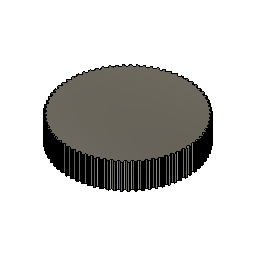
gear_75z (Autodesk Fusion 360 design; units mm, degrees)
Autodesk Fusion 360 part; units mm, degrees
sketch "Sketch1" plane through (0, 0, 0) normal (0, 0, 1) x (1, 0, 0) in component "gt2 pulley"
  circle A0 centre (0, 0) radius 23.8732 construction
  circle A1 centre (0, 0) radius 22.8692 construction
  line L0 (0, 0) -> (0, 23.8732) construction
  line L1 (0, 0) -> (0.9997, 23.8523) construction
  line L2 (0, 0) -> (1.4052, 23.8319) construction
  circle A2 centre (0, 0) radius 23.6192 construction
  arc A3 (0.3948, 23.4823) -> (0.4704, 23.1859) centre (1.3902, 23.5783) ccw
  circle A4 centre (0, 0) radius 23.4692 construction
  arc A5 (0.247, 23.6179) -> (0, 23.6192) centre (0, 0) ccw
  arc A6 (0.3948, 23.4823) -> (0.247, 23.6179) centre (0.2455, 23.468) ccw
  arc A7 (0.4704, 23.1859) -> (0.9577, 22.8492) centre (0.9809, 23.4037) ccw
  arc A8 (0, 23.6192) -> (-0.247, 23.6179) centre (0, 0) ccw
  arc A9 (-0.247, 23.6179) -> (-0.3948, 23.4823) centre (-0.2455, 23.468) ccw
  arc A10 (-0.4704, 23.1859) -> (-0.3948, 23.4823) centre (-1.3902, 23.5783) ccw
  arc A11 (-0.9577, 22.8492) -> (-0.4704, 23.1859) centre (-0.9809, 23.4037) ccw
  arc A12 (0.9577, 22.8492) -> (-0.9577, 22.8492) centre (0, 0) ccw
  point P0 (1.3902, 23.5783)
  point P1 (0, 23.6192)
  dimension "d18" = 47.7465
  dimension "d19" = 2.4
  dimension "d22" = 1.004
  dimension "d24" = 0.75
  dimension "d26" = 1
  dimension "d27" = 0.15
  dimension "d28" = 0.15
  dimension "d47" = 0.555
  dimension "d52" = 3.812
  constraint coincident A0.centre A1.centre
  constraint coincident A0 L0.end
  constraint vertical L0
  constraint coincident A0 L1.end
  constraint coincident A0 L2.end
  constraint concentric A1 A2
  constraint coincident A1 A7.end
  constraint coincident L1 A7.end
  constraint coincident A2 P0
  constraint coincident L2 P0
  constraint coincident P0 A3.centre
  constraint coincident A2 P1
  constraint coincident L0 P1
  constraint concentric A2 A4
  constraint coincident P1 A5.end
  constraint coincident A4 A6.centre
  constraint coincident A3.start A6.start
  constraint tangent A3 A6
  constraint tangent A3 A7
  constraint symmetric L0 A7.end A11.start
  constraint symmetric L0 A3.start A9.end
  constraint symmetric L0 A3.end A10.start
  constraint symmetric L0 A3 A10
  constraint symmetric L0 A5.start A8.end
  constraint symmetric L0 P1 A5.end
  constraint symmetric L0 A5 A8
  constraint symmetric L0 A6 A9
  constraint symmetric L0 A7 A11
  constraint coincident A1 A11.start
  constraint tangent A1 A7
  constraint coincident L1 A7.centre
  measures "d18" diameter of A0
  measures "d19" angle of L0 L1
  measures "d22" distance of A0 A1
  measures "d24" distance of A1 A2
  measures "d26" radius of A3
  measures "d27" distance of A2 A4
  measures "d28" radius of A6
  measures "d47" radius of A7
extrude "Extrude1" add sketch "Sketch1" along normal blind 10 makes body 1
pattern_circular "C-Pattern1" count 75 over 360 about axis through (0, 0, 1.75) along (0, 0, 1) of bodies 1 makes body 2 at (-2.655, 22.7146, 6.6667) makes body 3 at (-3.9188, 22.531, 6.6667) makes body 4 at (-6.4059, 21.9538, 6.6667) makes body 5 at (-7.6214, 21.5619, 6.6667) makes body 6 at (-9.9774, 20.578, 6.6667) makes body 7 at (-10.3587, 20.3887, 3.3333) makes body 8 at (-12.7442, 18.9892, 6.6667) makes body 9 at (-13.6138, 18.3757, 3.3333) makes body 10 at (-16.1898, 16.1522, 6.6667) makes body 11 at (-16.4877, 15.848, 3.3333) makes body 12 at (-18.2802, 13.7418, 6.6667) makes body 13 at (-18.8997, 12.8764, 3.3333) makes body 14 at (-20.2173, 10.6894, 6.6667) makes body 15 at (-21.1233, 8.764, 6.6667) makes body 16 at (-21.5082, 7.7717, 3.3333) makes body 17 at (-22.2891, 5.1185, 6.6667) makes body 18 at (-22.5031, 4.076, 3.3333) makes body 19 at (-22.8306, 1.3297, 6.6667) makes body 20 at (-22.8617, -0.5853, 6.6667) makes body 21 at (-22.7326, -2.4963, 6.6667) makes body 22 at (-22.5918, -3.5513, 6.6667) makes body 23 at (-21.9979, -6.2524, 6.6667) makes body 24 at (-21.1639, -8.6656, 6.6667) makes body 25 at (-20.6472, -9.8334, 6.6667) makes body 26 at (-19.5339, -11.8924, 6.6667) makes body 27 at (-19.1942, -12.4332, 3.3333) makes body 28 at (-18.0865, -13.9957, 3.3333) makes body 29 at (-16.2648, -16.0766, 6.6667) makes body 30 at (-14.3714, -17.7895, 6.6667) makes body 31 at (-12.8324, -18.9296, 6.6667) makes body 32 at (-12.4778, -19.1653, 3.3333) makes body 33 at (-9.4958, -20.8046, 6.6667) makes body 34 at (-9.1069, -20.9778, 3.3333) makes body 35 at (-7.3196, -21.6662, 3.3333) makes body 36 at (-5.4809, -22.2027, 3.3333) makes body 37 at (-3.6038, -22.5835, 6.6667) makes body 38 at (-0.8513, -22.8534, 6.6667) makes body 39 at (1.064, -22.8445, 6.6667) makes body 40 at (2.9718, -22.6753, 6.6667) makes body 41 at (4.8588, -22.3471, 6.6667) makes body 42 at (5.8933, -22.0969, 3.3333) makes body 43 at (8.5176, -21.2239, 6.6667) makes body 44 at (10.8303, -20.1422, 6.6667) makes body 45 at (12.4778, -19.1653, 6.6667) makes body 46 at (12.8324, -18.9296, 3.3333) makes body 47 at (14.8625, -17.3813, 6.6667) makes body 48 at (16.4137, -15.9246, 6.6667) makes body 49 at (18.0865, -13.9957, 6.6667) makes body 50 at (18.8396, -12.9642, 6.6667) makes body 51 at (19.4224, -12.0737, 3.3333) makes body 52 at (20.3645, -10.4061, 3.3333) makes body 53 at (21.4718, -7.8717, 6.6667) makes body 54 at (22.0552, -6.0474, 6.6667) makes body 55 at (22.444, -4.3898, 6.6667) makes body 56 at (22.7548, -2.2846, 6.6667) makes body 57 at (22.8662, -0.3725, 6.6667) makes body 58 at (22.8172, 1.5422, 6.6667) makes body 59 at (22.6955, 2.8135, 6.6667) makes body 60 at (22.0831, 5.9447, 6.6667) makes body 61 at (21.7168, 7.1681, 6.6667) makes body 62 at (21.3598, 8.1708, 3.3333) makes body 63 at (19.9109, 11.2498, 6.6667) makes body 64 at (18.8997, 12.8764, 6.6667) makes body 65 at (17.756, 14.4127, 6.6667) makes body 66 at (17.4846, 14.7408, 3.3333) makes body 67 at (15.5773, 16.7436, 6.6667) makes body 68 at (14.1216, 17.9884, 6.6667) makes body 69 at (13.2694, 18.6259, 3.3333) makes body 70 at (10.3587, 20.3887, 6.6667) makes body 71 at (9.9774, 20.578, 3.3333) makes body 72 at (7.4203, 21.6319, 6.6667) makes body 73 at (4.9628, 22.3243, 6.6667) makes body 74 at (3.0774, 22.6612, 6.6667) makes body 75 at (1.8076, 22.7977, 6.6667)
sketch "Sketch2" plane through (0, 0, 10) normal (0, 0, 1) x (-1, 0, 0)
  arc A0 (-9.9118, -21.2916) -> (-9.832, -21.4756) centre (-9.7696, -21.3392) ccw
  arc A1 (-9.832, -21.4756) -> (-9.3806, -21.6765) centre (0, 0) ccw
  arc A2 (-9.3806, -21.6765) -> (-9.1904, -21.6128) centre (-9.321, -21.5389) ccw
  arc A3 (-9.0008, -21.3727) -> (-9.1904, -21.6128) centre (-8.3201, -22.1053) ccw
  arc A4 (-8.4187, -21.2633) -> (-9.0008, -21.3727) centre (-8.623, -21.7793) ccw
  arc A5 (-10.1685, -20.4842) -> (-8.4187, -21.2633) centre (0, 0) ccw
  arc A6 (-9.8603, -20.9901) -> (-10.1685, -20.4842) centre (-10.4152, -20.9814) ccw
  arc A7 (-9.9118, -21.2916) -> (-9.8603, -20.9901) centre (-10.8602, -20.9744) ccw
  circle A8 centre (0, 0) radius 22.8692
  constraint concentric A1 A8
extrude "Extrude2" add sketch "Sketch2" against normal blind 10 contours A5 A8 bodies 1 2 3 4 5 6 7 8 9 10 11 12 13 14 15 16 17 18 19 20 21 22 23 24 25 26 27 28 29 30 31 32 33 34 35 36 37 38 39 40 41 42 43 44 45 46 47 48 49 50 51 52 53 54 55 56 57 58 59 60 61 62 63 64 65 66 67 68 69 70 71 72 73 74 75
extrude "Extrude4" [suppressed] in component "gt2 pulley"
pattern_circular "C-Pattern7" [suppressed] in component "gt2 pulley"
extrude "Extrude3" [suppressed] in component "gt2 pulley"
pattern_circular "C-Pattern6" [suppressed] in component "gt2 pulley"
extrude "Extrude2'" [suppressed] in component "gt2 pulley"
pattern_circular "C-Pattern5" [suppressed] in component "gt2 pulley"
extrude "Extrude1'" [suppressed] in component "gt2 pulley"
pattern_circular "C-Pattern4" [suppressed] in component "gt2 pulley"
pattern_circular "C-Pattern3" [suppressed] in component "gt2 pulley"
pattern_circular "C-Pattern2" [suppressed] in component "gt2 pulley"
pattern_circular "C-Pattern1'" [suppressed] in component "gt2 pulley"
copy_body "Body->Comp1" [suppressed] in component "Component"
copy_body "Body->Comp2" [suppressed] in component "Component'"
copy_body "Body->Comp3" [suppressed] in component "Component''"
copy_body "Body->Comp4" [suppressed] in component "Component'''"
copy_body "Body->Comp5" [suppressed] in component "Component''''"
copy_body "Body->Comp6" [suppressed] in component "Component'''''"
copy_body "Body->Comp7" [suppressed] in component "Component''''''"
copy_body "Body->Comp8" [suppressed] in component "Component'''''''"
copy_body "Body->Comp9" [suppressed] in component "Component''''''''"
copy_body "Body->Comp10" [suppressed] in component "Component'''''''''"
copy_body "Body->Comp11" [suppressed] in component "Component''''''''''"
copy_body "Body->Comp12" [suppressed] in component "Component'''''''''''"
copy_body "Body->Comp13" [suppressed] in component "Component''''''''''''"
copy_body "Body->Comp14" [suppressed] in component "Component'''''''''''''"
copy_body "Body->Comp15" [suppressed] in component "Component''''''''''''''"
copy_body "Body->Comp16" [suppressed] in component "Component'''''''''''''''"
copy_body "Body->Comp17" [suppressed] in component "Component''''''''''''''''"
copy_body "Body->Comp18" [suppressed] in component "Component'''''''''''''''''"
copy_body "Body->Comp19" [suppressed] in component "Component''''''''''''''''''"
copy_body "Body->Comp20" [suppressed] in component "Component'''''''''''''''''''"
component "gt2 pulley" placed x (1, 0, 0) y (0, 1, 0) z (0, 0, 1) at (0, 0, 0)
equation "NumTeeth = 75" comment "min 20"
equation "ToothPitch = 2 mm"
equation "PullyDia = NumTeeth * ToothPitch / PI"
equation "ToothAng = ( ( 360 / NumTeeth ) * 1 deg )"
equation "TransOffsetAngle = ToothAng * 0.2"
equation "Sholulder_Radius = 0.15 mm"
equation "Root_Radius = 0.555 mm"
equation "TransRadius = 1 mm"
equation "ToolHeight = 0.75 mm"
equation "PLD = 0.254 mm"
equation "d18 = PullyDia"
equation "d19 = ToothAng / 2"
equation "d22 = PLD + ToolHeight"
equation "d24 = ToolHeight"
equation "d26 = TransRadius"
equation "d27 = Sholulder_Radius"
equation "d31 = NumTeeth"
equation "d33 = NumTeeth"
equation "d35 = NumTeeth"
equation "d37 = NumTeeth"
equation "d41 = NumTeeth"
equation "d45 = NumTeeth"
equation "d47 = Root_Radius"
equation "d50 = NumTeeth"
